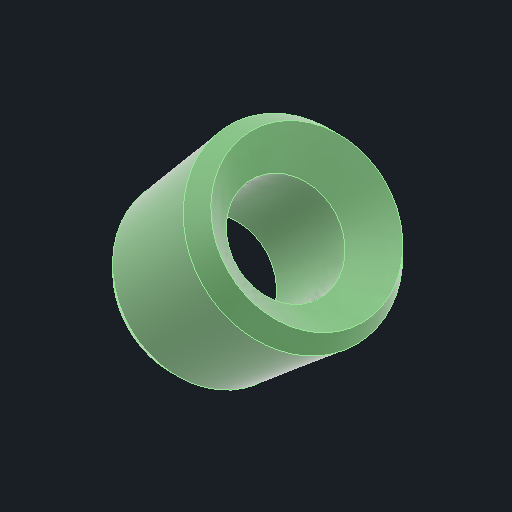
# Autodesk Inventor part: Roller
Saved by Autodesk Inventor 2023.1 (Build 271208000, 208)
## iProperties
Created: 2022-11-26
Part Number: Roller
Material: PC/ABS Plastic
Document SubType Name: Modeling
Designer: aubrey-work
Density: 0.357273 g/cm^3
Appearance: Smooth - Dark Forest Green
Author: aubrey-work
Autodesk Inventor part; units mm, degrees
ref_plane "YZ Plane" through (0, 0, 0) normal (1, 0, 0) x (0, 1, 0)
ref_plane "XZ Plane" through (0, 0, 0) normal (0, 1, 0) x (-1, 0, 0)
ref_plane "XY Plane" through (0, 0, 0) normal (0, 0, 1) x (1, 0, 0)
derived "Slew Bearing Master.ipt"
sketch "Sketch1" plane through (0, 0, 0) normal (0, 1, 0) x (-1, 0, 0)
  circle A0 centre (0, 0) radius 21.151
  ellipse E0 centre (-21.151, 0) end of major axis (-26.8785, 0) minor radius 4.05
  line L0 (-15.4234, 0) -> (-26.8785, 0)
  line L1 (-21.151, -4.05) -> (-21.151, 4.05)
  line L2 (0, 0) -> (-21.151, 0)
  line L3 (0, 0) -> (-19.6, -3.8987)
sketch "Sketch2" plane through (0, 0, 0) normal (0, 0, 1) x (1, 0, 0)
  line L0 (26.8785, 0) -> (15.4234, 0)
  line L1 (15.4234, 0) -> (21.151, -5.7276)
  line L2 (21.151, -5.7276) -> (26.8785, 0)
  line L3 (26.8785, 0) -> (21.151, 5.7276)
  line L4 (21.151, 5.7276) -> (15.4234, 0)
  line L5 (18.2872, 2.8638) -> (24.0148, -2.8638)
  line L6 (18.2872, -2.8638) -> (24.0148, 2.8638)
  line L7 (21.151, 5.7276) -> (21.151, -5.7276)
  line L8 (26.535, 0) -> (31.135, 0)
  line L9 (31.135, 0) -> (31.135, -5.7276)
  line L10 (31.135, -5.7276) -> (21.951, -5.7276)
  line L11 (21.951, -5.7276) -> (21.951, -4.9983)
  line L12 (21.951, -4.9983) -> (26.2422, -0.7071)
  arc A0 (26.2422, -0.7071) -> (26.535, 0) centre (25.535, 0) ccw
  arc A1 (26.535, 0) -> (26.2422, 0.7071) centre (25.535, 0) ccw
  line L13 (21.951, 4.9983) -> (26.2422, 0.7071)
  line L14 (21.951, 5.7276) -> (21.951, 4.9983)
  line L15 (31.135, 5.7276) -> (21.951, 5.7276)
  line L16 (31.135, 0) -> (31.135, 5.7276)
  line L17 (20.351, 5.7276) -> (20.351, 4.9983)
  line L18 (11.1669, 5.7276) -> (20.351, 5.7276)
  line L19 (20.351, 4.9983) -> (16.0598, 0.7071)
  line L20 (11.1669, 0) -> (11.1669, 5.7276)
  line L21 (11.1669, 0) -> (11.1669, -5.7276)
  arc A2 (16.0598, 0.7071) -> (15.7669, 0) centre (16.7669, 0) ccw
  arc A3 (15.7669, 0) -> (16.0598, -0.7071) centre (16.7669, 0) ccw
  line L22 (20.351, -4.9983) -> (16.0598, -0.7071)
  line L23 (15.7669, 0) -> (11.1669, 0)
  line L24 (20.351, -5.7276) -> (20.351, -4.9983)
  line L25 (11.1669, -5.7276) -> (20.351, -5.7276)
  line L26 (28.835, 5.7276) -> (28.835, -5.7276)
  line L27 (30.335, 5.7276) -> (30.335, -5.7276)
  line L28 (27.335, 5.7276) -> (27.335, -5.7276)
  line L29 (14.9669, 5.7276) -> (14.9669, -5.7276)
  line L30 (13.4669, 5.7276) -> (13.4669, -5.7276)
  line L31 (25.2622, 1.0506) -> (20.1004, -4.1113)
  line L32 (20.1004, -4.1113) -> (20.6553, -4.6662)
  line L33 (20.6553, -4.6662) -> (21.7981, -4.36)
  line L34 (21.7981, -4.36) -> (25.8359, -0.972)
  line L35 (25.8359, -0.972) -> (26.1421, 0.1708)
  line L36 (26.1421, 0.1708) -> (25.2622, 1.0506)
  line L37 (25.8359, -0.972) -> (22.123, -4.6849)
  line L38 (22.123, -4.6849) -> (21.7981, -4.36)
  point P0 (0, 0)
  point P1 (22.6813, -1.5303)
  point P2 (26.0963, 0)
  point P3 (24.2116, 0)
  point P4 (21.151, -3.0606)
  point P5 (21.151, -4.5334)
revolve "Revolution2" add sketch "Sketch2" angle 360 about axis through (18.2872, -2.8638, 0) along (0.7071068, 0.7071068, 0) contours L35 L34 L5 L31 L0 | L5 L34 L33 L7 L31
equation "\"gap\" = 0.1"
equation "\"airgap\" = 0.4"
equation "\"wallgap\" = 0.8"
equation "\"roller_outerDiameter\" = 8"
equation "\"roller_diameter\" = 8"
equation "\"bolt_diameter\" = 3"
equation "\"outerBolt_diameter\" = 3"
equation "\"innerBolt_diameter\" = 3"
equation "\"elephantsFoot\" = 0.4"
